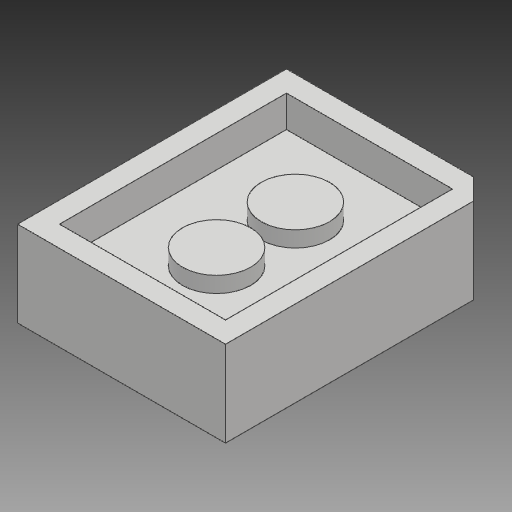
# Autodesk Inventor part: AEDR-8300-1Wx Encoder
Saved by Autodesk Inventor 2019.4 (Build 234330000, 330)
## iProperties
Part Number: AEDR-8300-1Wx Encoder
Material: Generisch
Document SubType Name: Modeling
Designer: rYan
Density: 1 g/cm^3
Appearance: Vorgabe
Mass: 0.0255238 g
Surface Area: 0.810357 cm^2
Volume: 0.0255238 cm^3
Author: rYan
Autodesk Inventor part; units mm, degrees
ref_plane "YZ Plane" through (0, 0, 0) normal (1, 0, 0) x (0, 1, 0)
ref_plane "XZ Plane" through (0, 0, 0) normal (0, 1, 0) x (-1, 0, 0)
ref_plane "XY Plane" through (0, 0, 0) normal (0, 0, 1) x (1, 0, 0)
sketch "Skizze1" plane through (0, 0, 0) normal (0, 0, 1) x (1, 0, 0)
  line L0 (-1.98, -2.56) -> (1.98, -2.56)
  line L1 (1.98, -2.56) -> (1.98, 2.56)
  line L2 (1.98, 2.56) -> (-1.98, 2.56)
  line L3 (-1.98, 2.56) -> (-1.98, -2.56)
  line L4 (-1.98, -2.56) -> (1.98, 2.56) construction
  line L5 (1.98, -2.56) -> (-1.98, 2.56) construction
  point P0 (0, 0)
  dimension "d0" = 3.96
  dimension "d1" = 5.12
  constraints: 12 end point, 2 midpoint, 2 parallel, 1 horizontal, 1 perpendicular
  measures "d0" distance of L2.end L1.end
  measures "d1" distance of L1.end L0.end
extrude "Extrusion1" add sketch "Skizze1" along normal blind 1.63
sketch "Skizze2" plane through (0, 0, 1.63) normal (0, 0, 1) x (1, 0, 0)
  line L0 (-1.98, -2.56) -> (1.98, -2.56) projected
  line L1 (1.98, -2.56) -> (1.98, 2.56) projected
  line L2 (1.98, 2.56) -> (-1.98, 2.56) projected
  line L3 (-1.98, 2.56) -> (-1.98, -2.56) projected
  line L4 (-1.58, -2.16) -> (1.58, -2.16)
  line L5 (1.58, -2.16) -> (1.58, 2.16)
  line L6 (1.58, 2.16) -> (-1.58, 2.16)
  line L7 (-1.58, 2.16) -> (-1.58, -2.16)
  line L8 (-1.58, -2.16) -> (1.58, 2.16) construction
  line L9 (1.58, -2.16) -> (-1.58, 2.16) construction
  point P0 (0, 0)
  dimension "d4" = 0.4
  dimension "d5" = 0.4
  constraints: 12 end point, 2 midpoint, 2 parallel, 1 horizontal, 1 perpendicular
  measures "d4" distance between parallel lines of L2 L6
  measures "d5" distance between parallel lines of L3 L7
extrude "Extrusion2" cut sketch "Skizze2" against normal blind 0.6 contours L7 L6 L5 L4
sketch "Skizze3" plane through (0, 0, 1.03) normal (0, 0, 1) x (1, 0, 0)
  line L0 (0, 3.584) -> (0, -3.584) projected
  circle A0 centre (0, 0.75) radius 0.65
  circle A1 centre (0, -0.75) radius 0.65
  line L1 (-2.772, 0) -> (2.772, 0) projected
  point P0 (0, 0)
  dimension "d8" = 1.3
  dimension "d9" = 1.3
  dimension "d10" = 1.5
  constraints: 2 centre point, 2 point on line, 1 symmetric about line
  measures "d8" diameter of A0
  measures "d9" diameter of A1
  measures "d10" distance of A1.centre A0.centre
extrude "Extrusion3" add sketch "Skizze3" along normal blind 0.3
chamfer "Fase1" distance 0.4 angle 45 1 edges at (1.98, 2.56, 0.815)
equation "\"d9\" = d8"
